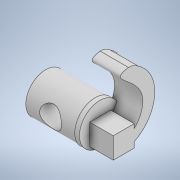
# Autodesk Inventor part: Part13
Saved by Autodesk Inventor 2020.2 (Build 242310000, 310)
## iProperties
Created: 2020-03-26
Part Number: Part13
Material: Generic
Document SubType Name: Modeling
Designer: iamin
Density: 1 g/cm^3
Appearance: Default
Author: iamin
Autodesk Inventor part; units mm, degrees
ref_plane "YZ Plane" through (0, 0, 0) normal (1, 0, 0) x (0, 1, 0)
ref_plane "XZ Plane" through (0, 0, 0) normal (0, 1, 0) x (-1, 0, 0)
ref_plane "XY Plane" through (0, 0, 0) normal (0, 0, 1) x (1, 0, 0)
sketch "Sketch1" plane through (0, 0, 0) normal (1, 0, 0) x (0, 1, 0)
  circle A0 centre (0, 0) radius 8.45
  dimension "d0" = 16.9
  constraints: 1 centre point, 1 coincident
  measures "d0" diameter of A0
extrude "Extrusion1" add sketch "Sketch1" along normal mid plane 21
sketch "Sketch2" plane through (10.5, 0, 0) normal (1, 0, 0) x (0, 0, -1)
  circle A0 centre (0, 0) radius 7.725
  circle A1 centre (0, 0) radius 9.725
  dimension "d3" = 2
  dimension "d4" = 19.45
  constraints: 2 centre point, 2 coincident
  measures "d3" radial gap between concentric circles of A0 A1
  measures "d4" diameter of A1
extrude "Extrusion2" cut sketch "Sketch2" against normal blind 21.5 contours A0
sketch "Sketch3" plane through (0, 0, 0) normal (0, 0, 1) x (1, 0, 0)
  circle A0 centre (0, 0) radius 5.625
  dimension "d7" = 11.25
  constraints: 1 centre point, 1 coincident
  measures "d7" diameter of A0
extrude "Extrusion3" add sketch "Sketch3" along normal mid plane 18
sketch "Sketch4" plane through (0, 0, 0) normal (0, 0, 1) x (1, 0, 0)
  circle A0 centre (0, 0) radius 4.625
  dimension "d10" = 9.25
  constraints: 1 centre point, 1 coincident
  measures "d10" diameter of A0
extrude "Extrusion5" cut sketch "Sketch4" along normal mid plane 100
sketch "Sketch5" plane through (10.5, 0, 0) normal (1, 0, 0) x (0, 0, -1)
  circle A0 centre (0, 0) radius 8.675
  dimension "d15" = 17.35
  constraints: 1 centre point, 1 coincident
  measures "d15" diameter of A0
extrude "Extrusion6" add sketch "Sketch5" along normal blind 2
sketch "Sketch6" plane through (12.5, 0, 0) normal (1, 0, 0) x (0, 0, -1)
  arc A0 (1.0628, -4.9847) -> (6.3756, 23.0304) centre (-2.1717, 10.14) ccw
  spline S0 degree 4 poles (1.0628, -0.783) (3.325, -0.3237) (6.6509, 1.9196) (12.5543, 12.8577) (0.0955, 21.0445) (-3.8878, 23.6903) (2.1134, 24.7257) knots 0 0 0 0 0 0.38125 0.63125 1 1 1 1 1
  line L0 (-1.8785, -1.3802) -> (4.0041, -0.1858) construction
  arc A1 (-1.2523, -0.8951) -> (3.2382, 0.0167) centre (-0.4606, 6.7196) ccw construction
  spline S1 degree 2 poles (6.3756, 23.0304) (3.3857, 25.3291) (1.0628, 24.5204) knots 0 0 0 1 1 1
  line L1 (-6.8176, 23.1848) -> (11.0445, 26.2665) construction
  arc A2 (9.1477, 24.9445) -> (-4.5875, 22.5748) centre (6.4085, -0.169) ccw construction
  line L2 (-4.3138, 2.8134) -> (4.5692, 2.8134)
  line L3 (4.5692, -6.1723) -> (-4.3138, -6.1723)
  line L4 (-4.3138, -6.1723) -> (-4.3138, 2.8134)
  line L5 (4.5692, 2.8134) -> (4.5692, 1.038)
  line L6 (4.5692, -3.7804) -> (4.5692, -6.1723)
  point P0 (0, 0)
  point P1 (-0.6365, 21.8121)
  point P2 (1.0628, -0.783)
  point P3 (3.2364, 24.6304)
  point P4 (2.1134, 24.7257)
  point P5 (2.1133, 24.7254)
  point P6 (1.0633, 24.5166)
  constraints: 14 end point, 6 point on circle, 4 midpoint, 3 centre point, 3 parallel, 2 perpendicular, 1 horizontal, 16 other
extrude "Extrusion7" add sketch "Sketch6" along normal blind 10 and the other way blind 2
sketch "Sketch7" plane through (-10.5, 0, 0) normal (-1, 0, 0) x (0, 0, 1)
  circle A0 centre (0, 0) radius 8.45
  circle A1 centre (0, 0) radius 11.1999
  dimension "d23" = 16.9
  constraints: 2 centre point, 2 coincident
  measures "d23" diameter of A0
extrude "Extrusion8" cut sketch "Sketch7" against normal blind 17.75
body "Solid1"
